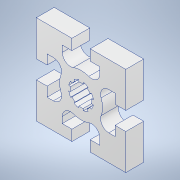
# Autodesk Inventor part: Perfil-de-aluminio-0001-002
Saved by Autodesk Inventor 2020.1 (Build 241239000, 239)
## iProperties
Created: 2024-04-15
Part Number: Perfil-de-aluminio-0001-002
Material: Aluminum 6061
Document SubType Name: Modeling
Designer: MiguelBarbosa
Density: 2.7 g/cm^3
Appearance: Aluminum - Flat
Author: MiguelBarbosa
Autodesk Inventor part; units mm, degrees
ref_plane "YZ Plane" through (0, 0, 0) normal (1, 0, 0) x (0, 1, 0)
ref_plane "XZ Plane" through (0, 0, 0) normal (0, 1, 0) x (-1, 0, 0)
ref_plane "XY Plane" through (0, 0, 0) normal (0, 0, 1) x (1, 0, 0)
sketch "Sketch2" plane through (0, 0, 0) normal (0, 0, 1) x (1, 0, 0)
  line L0 (0, 0) -> (0, 6) construction
  circle A0 centre (0, 0) radius 6 construction
  circle A1 centre (0, 0) radius 7 construction
  arc A2 (1.1705, 5.8847) -> (-1.1705, 5.8847) centre (0, 0) ccw
  line L1 (-1.3656, 6.8655) -> (0, 0) construction
  line L2 (-1.3656, 6.8655) -> (-1.1705, 5.8847)
  arc A3 (-1.3656, 6.8655) -> (-3.889, 5.8203) centre (0, 0) ccw
  line L3 (0, 0) -> (-3.889, 5.8203) construction
  line L4 (-3.889, 5.8203) -> (-3.3334, 4.9888)
  line L5 (-6.8655, 1.3656) -> (-5.8847, 1.1705)
  arc A4 (-5.8203, 3.889) -> (-6.8655, 1.3656) centre (0, 0) ccw
  line L6 (-5.8203, 3.889) -> (-4.9888, 3.3334)
  arc A5 (-3.3334, 4.9888) -> (-4.9888, 3.3334) centre (0, 0) ccw
  line L7 (-5.8203, -3.889) -> (-4.9888, -3.3334)
  arc A6 (-6.8655, -1.3656) -> (-5.8203, -3.889) centre (0, 0) ccw
  line L8 (-6.8655, -1.3656) -> (-5.8847, -1.1705)
  arc A7 (-5.8847, 1.1705) -> (-5.8847, -1.1705) centre (0, 0) ccw
  line L9 (-1.3656, -6.8655) -> (-1.1705, -5.8847)
  arc A8 (-3.889, -5.8203) -> (-1.3656, -6.8655) centre (0, 0) ccw
  line L10 (-3.889, -5.8203) -> (-3.3334, -4.9888)
  arc A9 (-4.9888, -3.3334) -> (-3.3334, -4.9888) centre (0, 0) ccw
  line L11 (3.889, -5.8203) -> (3.3334, -4.9888)
  arc A10 (1.3656, -6.8655) -> (3.889, -5.8203) centre (0, 0) ccw
  line L12 (1.3656, -6.8655) -> (1.1705, -5.8847)
  arc A11 (-1.1705, -5.8847) -> (1.1705, -5.8847) centre (0, 0) ccw
  line L13 (6.8655, -1.3656) -> (5.8847, -1.1705)
  arc A12 (5.8203, -3.889) -> (6.8655, -1.3656) centre (0, 0) ccw
  line L14 (5.8203, -3.889) -> (4.9888, -3.3334)
  arc A13 (3.3334, -4.9888) -> (4.9888, -3.3334) centre (0, 0) ccw
  line L15 (5.8203, 3.889) -> (4.9888, 3.3334)
  arc A14 (6.8655, 1.3656) -> (5.8203, 3.889) centre (0, 0) ccw
  line L16 (6.8655, 1.3656) -> (5.8847, 1.1705)
  arc A15 (5.8847, -1.1705) -> (5.8847, 1.1705) centre (0, 0) ccw
  line L17 (1.3656, 6.8655) -> (1.1705, 5.8847)
  arc A16 (3.889, 5.8203) -> (1.3656, 6.8655) centre (0, 0) ccw
  line L18 (3.889, 5.8203) -> (3.3334, 4.9888)
  arc A17 (4.9888, 3.3334) -> (3.3334, 4.9888) centre (0, 0) ccw
  circle A18 centre (0, 0) radius 12
  line L19 (-20.9, 20.9) -> (-14.1, 20.9) construction
  line L20 (-14.1, 20.9) -> (-14.1, 14.1) construction
  line L21 (-14.1, 14.1) -> (-20.9, 14.1) construction
  line L22 (-20.9, 14.1) -> (-20.9, 20.9) construction
  line L23 (-20.9, 20.9) -> (-14.1, 14.1) construction
  line L24 (-14.1, 20.9) -> (-20.9, 14.1) construction
  line L25 (-21.5, 13.5) -> (-13.5, 13.5) construction
  line L26 (-13.5, 13.5) -> (-13.5, 21.5) construction
  line L27 (-13.5, 21.5) -> (-21.5, 21.5) construction
  line L28 (-21.5, 21.5) -> (-21.5, 13.5) construction
  line L29 (-21.5, 13.5) -> (-13.5, 21.5) construction
  line L30 (-13.5, 13.5) -> (-21.5, 21.5) construction
  line L31 (-19, 20.9) -> (-16, 20.9)
  line L32 (-19, 20.9) -> (-19, 21.5)
  line L33 (-25, 25) -> (-25, 5.1)
  line L34 (-25, 25) -> (-5.1, 25)
  line L35 (-25, 5.1) -> (-19, 5.1)
  line L36 (-19, 5.1) -> (-19, 10.5)
  line L37 (-19, 10.5) -> (-12, 10.5) construction
  line L38 (-12, 0) -> (-12, 10.5) construction
  arc A19 (-11.2123, 4.276) -> (-15.5, 10.5) centre (-15.5, 5.9111) ccw
  line L39 (-19, 10.5) -> (-15.5, 10.5)
  line L40 (-5.1, 25) -> (-5.1, 19)
  line L41 (-5.1, 19) -> (-10.5, 19)
  line L42 (-10.5, 19) -> (-10.5, 15.5)
  arc A20 (-10.5, 15.5) -> (-4.276, 11.2123) centre (-5.9111, 15.5) ccw
  point P0 (-4.2426, 4.2426)
  point P1 (-6, 0)
  point P2 (-4.2426, -4.2426)
  point P3 (0, -6)
  point P4 (4.2426, -4.2426)
  point P5 (6, 0)
  point P6 (4.2426, 4.2426)
  point P7 (-5.8847, 1.1705)
  point P8 (-3.3334, 4.9888)
  point P9 (1.1705, 5.8847)
  point P10 (4.9888, 3.3334)
  point P11 (-1.1705, -5.8847)
  point P12 (-4.9888, -3.3334)
  point P13 (-17.5, 17.5)
  point P14 (-17.5, 20.9)
  dimension "d1" = 14
  dimension "d2" = 12
  dimension "d7" = 360
  dimension "d10" = 22.5
  dimension "d11" = 24
  dimension "d14" = 17.5
  dimension "d15" = 17.5
  dimension "d16" = 6.8
  dimension "d17" = 8
  dimension "d18" = 3
  dimension "d19" = 25
  dimension "d20" = 5.1
  dimension "d21" = 25
  dimension "d22" = 6
  dimension "d23" = 3
  constraints: 86 end point, 45 point on circle, 21 centre point, 7 horizontal, 7 midpoint, 7 perpendicular, 7 vertical, 6 coincident, 5 tangent, 4 parallel, 3 point on line, 1 collinear, 1 horizontal alignment, 97 other
  measures "d1" diameter of A1
  measures "d2" diameter of A0
  measures "d10" angle of L3 L1
  measures "d11" diameter of A18
  measures "d14" horizontal distance of point (0, 0) point (-17.5, 17.5)
  measures "d15" horizontal distance of point (0, 0) point (-17.5, 17.5)
  measures "d16" distance of L19.start L19.end
  measures "d17" distance of L26.end L27.end
  measures "d18" distance of L31.start L31.end
  measures "d19" distance from line of point (0, 0) L33
  measures "d20" vertical distance of point (0, 0) L33.end
  measures "d21" horizontal distance of L33.start point (0, 0)
  measures "d22" distance of L33.end L35.end
  measures "d23" distance from line of L25 L36.end
extrude "Extrusion1" add sketch "Sketch2" along normal blind 10 contours A18
extrude "Extrusion2" add sketch "Sketch2" along normal blind 10 contours A18 A19 L39 L36 L35 L33 L34 L40 L41 L42 A20
pattern_circular "Circular Pattern2" count 4 over 360 about axis through (0, 0, 0) along (0, 0, 1) of "Extrusion2"
equation "\"d15\" = d14"
equation "\"d21\" = d19"
body "Solid1"
